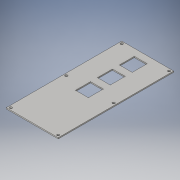
# Autodesk Inventor part: Cover Rev 4
Saved by Autodesk Inventor 2016 (Build 200138000, 138)
## iProperties
Created: 2018-02-03
Part Number: Cover Rev 4
Material: Generic
Document SubType Name: Modeling
Designer: Mom
Density: 1 g/cm^3
Appearance: Default
Author: Mom
Autodesk Inventor part; units mm, degrees
ref_plane "YZ Plane" through (0, 0, 0) normal (1, 0, 0) x (0, 1, 0)
ref_plane "XZ Plane" through (0, 0, 0) normal (0, 1, 0) x (-1, 0, 0)
ref_plane "XY Plane" through (0, 0, 0) normal (0, 0, 1) x (1, 0, 0)
sketch "Sketch1" plane through (0, 0, 0) normal (0, 1, 0) x (-1, 0, 0)
  line L0 (0, 0) -> (0, -200)
  line L1 (0, -200) -> (90, -200)
  line L2 (90, -200) -> (90, 0)
  line L3 (90, 0) -> (0, 0)
  line L4 (45, -200) -> (45, -188)
  line L5 (45, -188) -> (56.125, -188)
  line L6 (56.125, -188) -> (56.125, -162)
  line L7 (56.125, -162) -> (33.875, -162)
  line L8 (33.875, -162) -> (33.875, -188)
  line L9 (33.875, -188) -> (45, -188)
  line L10 (45, -150) -> (56.125, -150)
  line L11 (56.125, -150) -> (56.125, -124)
  line L12 (56.125, -124) -> (33.875, -124)
  line L13 (33.875, -124) -> (33.875, -150)
  line L14 (33.875, -150) -> (45, -150)
  line L15 (45, -112) -> (56.125, -112)
  line L16 (56.125, -112) -> (56.125, -86)
  line L17 (56.125, -86) -> (33.875, -86)
  line L18 (33.875, -86) -> (33.875, -112)
  line L19 (33.875, -112) -> (45, -112)
  circle A0 centre (86, -4) radius 2.1
  circle A1 centre (86, -100) radius 2.1
  circle A2 centre (86, -196) radius 2.1
  circle A3 centre (4, -4) radius 2.1
  circle A4 centre (4, -100) radius 2.1
  circle A5 centre (4, -196) radius 2.1
  dimension "d0" = 200
  dimension "d1" = 90
  dimension "d2" = 200
  dimension "d3" = 12
  dimension "d4" = 11.125
  dimension "d5" = 26
  dimension "d6" = 22.25
  dimension "d7" = 26
  dimension "d9" = 11.125
  dimension "d10" = 26
  dimension "d11" = 22.25
  dimension "d12" = 26
  dimension "d14" = 11.125
  dimension "d15" = 26
  dimension "d16" = 22.25
  dimension "d17" = 26
  dimension "d23" = 4.2
  dimension "d25" = 4.2
  constraints: 40 end point, 10 point on line, 6 centre point, 6 perpendicular, 2 vertical, 1 midpoint
  measures "d0" distance of L0.start L0.end
  measures "d1" distance of L0.end L1.end
  measures "d2" distance of L1.end L2.end
  measures "d3" distance of L4.start L4.end
  measures "d4" distance of L4.end L5.end
  measures "d5" distance of L5.end L6.end
  measures "d6" distance of L6.end L7.end
  measures "d7" distance of L7.end L8.end
  measures "d9" distance of L10.start L10.end
  measures "d10" distance of L10.end L11.end
  measures "d11" distance of L11.end L12.end
  measures "d12" distance of L12.end L13.end
  measures "d14" distance of L15.start L15.end
  measures "d15" distance of L15.end L16.end
  measures "d16" distance of L16.end L17.end
  measures "d17" distance of L17.end L18.end
  measures "d23" diameter of A0
  measures "d25" diameter of A2
extrude "Extrusion1" add sketch "Sketch1" against normal blind 2
body "Solid1"
